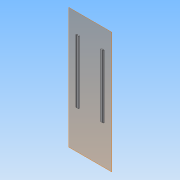
# Autodesk Inventor part: HOT SideBorder
Saved by Autodesk Inventor 2013 (Build 170138000, 138)
## iProperties
Created: 2018-07-29
Part Number: HOT SideBorder
Material: Generic
Document SubType Name: Modeling
Designer: Jeff Vyduna
Density: 1 g/cm^3
Author: Jeff Vyduna
Autodesk Inventor part; units mm, degrees
ref_plane "YZ Plane" through (0, 0, 0) normal (1, 0, 0) x (0, 1, 0)
ref_plane "XZ Plane" through (0, 0, 0) normal (0, 1, 0) x (-1, 0, 0)
ref_plane "XY Plane" through (0, 0, 0) normal (0, 0, 1) x (1, 0, 0)
ref_plane "Work Plane1" through (0, 0, 0) normal (0, 0, 1) x (1, 0, 0)
sketch "Sketch1" plane through (0, 0, 0) normal (0, 0, 1) x (1, 0, 0)
  line L0 (-452.8602, 908.0528) -> (-452.8602, -475.1907) projected
  line L1 (156.7398, -475.1907) -> (156.7398, 908.0528) projected
  line L2 (-452.8602, 908.0528) -> (-389.3602, 908.0528)
  line L3 (-389.3602, 908.0528) -> (-389.3602, -475.1907)
  line L4 (-389.3602, -475.1907) -> (-452.8602, -475.1907)
  line L5 (-452.8602, -475.1907) -> (-452.8602, 908.0528)
  line L6 (156.7398, 908.0528) -> (93.2398, 908.0528)
  line L7 (93.2398, 908.0528) -> (93.2398, -475.1907)
  line L8 (93.2398, -475.1907) -> (156.7398, -475.1907)
  line L9 (156.7398, -475.1907) -> (156.7398, 908.0528)
  point P0 (0, 0)
  dimension "borderW" = 63.5
  dimension "d1" = 63.5
  constraints: 16 end point, 4 parallel, 2 horizontal, 2 perpendicular, 1 collinear, 1 point on line
  measures "borderW" distance of L3.end L4.end
  measures "d1" distance of L8.end L7.end
extrude "Extrusion1" add sketch "Sketch1" along normal blind 19.05
sketch "Sketch2" plane through (0, 0, 19.05) normal (0, 0, 1) x (1, 0, 0)
  line L0 (-452.8602, 908.0528) -> (-452.8602, -475.1907) projected
  line L1 (-452.8602, -475.1907) -> (-389.3602, -475.1907) projected
  line L2 (-389.3602, 908.0528) -> (-452.8602, 908.0528) projected
  line L3 (156.7398, 908.0528) -> (93.2398, 908.0528) projected
  line L4 (93.2398, 908.0528) -> (93.2398, -475.1907) projected
  line L5 (93.2398, -475.1907) -> (156.7398, -475.1907) projected
  line L6 (156.7398, -475.1907) -> (156.7398, 908.0528) projected
  line L7 (-440.1602, 908.0528) -> (-427.9682, 908.0528)
  line L8 (-427.9682, 908.0528) -> (-427.9682, -475.1907)
  line L9 (-427.9682, -475.1907) -> (-440.1602, -475.1907)
  line L10 (-440.1602, -475.1907) -> (-440.1602, 908.0528)
  line L11 (144.0398, 908.0528) -> (131.8478, 908.0528)
  line L12 (131.8478, 908.0528) -> (131.8478, -475.1907)
  line L13 (131.8478, -475.1907) -> (144.0398, -475.1907)
  line L14 (144.0398, -475.1907) -> (144.0398, 908.0528)
  point P0 (0, 0)
  dimension "bRopeChannel" = 12.192
  dimension "d5" = 12.192
  dimension "d6" = 12.7
  dimension "d7" = 12.7
  constraints: 16 end point, 4 parallel, 2 collinear, 2 horizontal, 2 perpendicular, 2 point on line
  measures "bRopeChannel" distance of L8.end L9.end
  measures "d5" distance of L13.end L12.end
  measures "d6" distance between parallel lines of L0 L10
  measures "d7" distance between parallel lines of L14 L6
extrude "Extrusion2" cut sketch "Sketch2" against normal blind 12.7 contours L2 L8 L1 L10 | L14 L5 L12 L3
equation "\"d1\" = borderW"
equation "\"d5\" = bRopeChannel"
equation "\"d7\" = d6"
body "Solid1"
